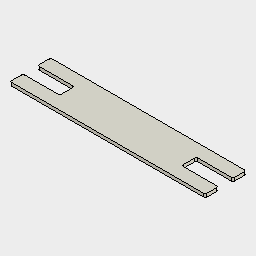
Acrylic Slide Holder (Autodesk Fusion 360 design; units mm, degrees)
Autodesk Fusion 360 part; units mm, degrees
sketch "Sketch1" plane through (0, 0, 0) normal (0, 0, 1) x (1, 0, 0)
  line L0 (-60, 12.5) -> (60, 12.5)
  line L1 (60, 12.5) -> (60, 4.5)
  line L2 (60, 4.5) -> (-60, 4.5)
  line L3 (-60, 4.5) -> (-60, 12.5)
  line L4 (-60, -4.5) -> (60, -4.5)
  line L5 (60, -4.5) -> (60, -12.5)
  line L6 (60, -12.5) -> (-60, -12.5)
  line L7 (-60, -12.5) -> (-60, -4.5)
  line L8 (-37.5, 4.5) -> (37.5, 4.5)
  line L9 (37.5, 4.5) -> (37.5, -4.5)
  line L10 (37.5, -4.5) -> (-37.5, -4.5)
  line L11 (-37.5, -4.5) -> (-37.5, 4.5)
  dimension "d24" = 120
  dimension "d25" = 8
  dimension "d26" = 8
  dimension "d27" = 25
  dimension "d28" = 75
  dimension "d34" = 60
  dimension "d35" = 12.5
  dimension "d38" = 37.5
  measures "d24" distance of L0.start L0.end
  measures "d25" distance of L0.start L2.end
  measures "d26" distance of L4.start L6.end
  measures "d27" distance of L0 L6
  measures "d28" distance of L8.start L8.end
  measures "d34" distance of origin L3
  measures "d35" distance of origin L0
  measures "d38" distance of origin L9
extrude "Extrude1" add sketch "Sketch1" along normal blind 2
fillet "Fillet1" radius 1 12 edges at (-60, 12.5, 1) (-60, 4.5, 1) (-60, -4.5, 1) (-60, -12.5, 1) (-37.5, 4.5, 1) (-37.5, -4.5, 1) (60, -12.5, 1) (60, -4.5, 1) (37.5, 4.5, 1) (37.5, -4.5, 1) (60, 4.5, 1) (60, 12.5, 1)
equation "d26 = d25"
equation "d34 = d24 / 2"
equation "d35 = d27 / 2"
equation "d38 = d28 / 2"
